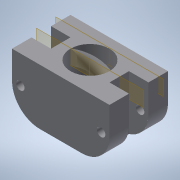
# Autodesk Inventor part: ScrewActuatorGripperCenter
Saved by Autodesk Inventor 2020.1 (Build 241239000, 239)
## iProperties
Created: 2016-10-15
Part Number: ScrewActuatorGripperCenter
Material: Generic
Document SubType Name: Modeling
Designer: Bardo91
Density: 1 g/cm^3
Appearance: Default
Author: Bardo91
Autodesk Inventor part; units mm, degrees
ref_plane "YZ Plane" through (0, 0, 0) normal (1, 0, 0) x (0, 1, 0)
ref_plane "XZ Plane" through (0, 0, 0) normal (0, 1, 0) x (-1, 0, 0)
ref_plane "XY Plane" through (0, 0, 0) normal (0, 0, 1) x (1, 0, 0)
sketch "Sketch1" plane through (0, 0, 0) normal (0, 0, 1) x (1, 0, 0)
  line L0 (0, 0) -> (0, 7)
  line L1 (0, 7) -> (7, 7)
  line L2 (7, 7) -> (7, 0)
  line L3 (7, 0) -> (14, 0)
  line L4 (14, 0) -> (14, 7)
  line L5 (14, 7) -> (21, 7)
  line L6 (21, 7) -> (21, 0)
  line L7 (21, 0) -> (28, 0)
  line L8 (28, 0) -> (28, -7)
  line L9 (28, -7) -> (21, -7)
  line L10 (21, -7) -> (21, -14)
  line L11 (21, -14) -> (28, -14)
  line L12 (28, -14) -> (28, -21)
  line L13 (28, -21) -> (21, -21)
  line L14 (21, -21) -> (21, -28)
  line L15 (21, -28) -> (14, -28)
  line L16 (14, -28) -> (14, -21)
  line L17 (14, -21) -> (7, -21)
  line L18 (7, -21) -> (7, -28)
  line L19 (7, -28) -> (0, -28)
  line L20 (0, -28) -> (0, -21)
  line L21 (0, -21) -> (-7, -21)
  line L22 (-7, -21) -> (-7, -14)
  line L23 (-7, -14) -> (0, -14)
  line L24 (0, -14) -> (0, -7)
  line L25 (0, -7) -> (-7, -7)
  line L26 (-7, -7) -> (-7, 0)
  line L27 (-7, 0) -> (0, 0)
  dimension "d55" = 7
  dimension "d56" = 7
  dimension "d57" = 7
  dimension "d58" = 7
  dimension "d59" = 7
  dimension "d60" = 7
  dimension "d61" = 7
  dimension "d62" = 90
  dimension "d63" = 7
  dimension "d64" = 7
  dimension "d65" = 90
  dimension "d66" = 7
  dimension "d67" = 7
  dimension "d68" = 7
  dimension "d69" = 7
  dimension "d70" = 7
  dimension "d71" = 7
  dimension "d72" = 7
  dimension "d73" = 7
  dimension "d74" = 7
  dimension "d75" = 7
  dimension "d76" = 7
  dimension "d77" = 90
  dimension "d93" = 7
  constraints: 56 end point, 15 perpendicular, 13 point on line, 3 horizontal, 2 vertical
  measures "d55" distance of L0.start L0.end
  measures "d56" distance of L0.end L1.end
  measures "d57" distance of L2.end L3.end
  measures "d58" distance of L3.end L4.end
  measures "d59" distance of L4.end L5.end
  measures "d60" distance of L6.end L7.end
  measures "d61" distance of L7.end L8.end
  measures "d62" angle of L7 L8
  measures "d63" distance of L8.end L9.end
  measures "d64" distance of L9.end L10.end
  measures "d65" angle of L10 L9
  measures "d66" distance of L10.end L11.end
  measures "d67" distance of L11.end L12.end
  measures "d68" distance of L13.end L14.end
  measures "d69" distance of L14.end L15.end
  measures "d70" distance of L16.end L17.end
  measures "d71" distance of L18.end L19.end
  measures "d72" distance of L19.end L20.end
  measures "d73" distance of L20.end L21.end
  measures "d74" distance of L21.end L22.end
  measures "d75" distance of L23.end L24.end
  measures "d76" distance of L24.end L25.end
  measures "d77" angle of L25 L24
  measures "d93" distance of L25.end L26.end
extrude "Extrusion1" add sketch "Sketch1" along normal blind 20
sketch "Sketch6" plane through (0, 0, 20) normal (0, 0, 1) x (1, 0, 0)
  line L0 (14, 0) -> (7, 0) projected
  line L1 (10.5, 0) -> (10.5, -21)
  line L2 (7, -21) -> (14, -21) projected
  circle A0 centre (10.5, -10.5) radius 7
  point P0 (0, 0)
  dimension "d94" = 14
  constraints: 3 midpoint, 2 end point, 1 centre point
  measures "d94" diameter of A0
extrude "Extrusion6" cut sketch "Sketch6" against normal through all
sketch "Sketch7" plane through (-7, -21, 0) normal (0, -1, 0) x (1, 0, 0)
  line L0 (0, 0) -> (0, 10)
  line L1 (0, 0) -> (0, 20) projected
  line L2 (0, 10) -> (3, 10)
  circle A0 centre (3, 10) radius 1.5
  point P0 (7, 0)
  dimension "d83" = 3
  dimension "d84" = 3
  constraints: 4 end point, 1 centre point, 1 coincident, 1 horizontal, 1 midpoint
  measures "d83" distance of L0.end L2.end
  measures "d84" diameter of A0
extrude "Extrusion7" cut sketch "Sketch7" against normal through all
pattern_circular "Circular Pattern3" count 4 over 360 about axis through (10.5, -10.5, 20) along (0, 0, -1) of "Extrusion7"
ref_plane "Work Plane3" through (10.5, -10.5, 20) normal (0, -1, 0) x (1, 0, 0)
ref_plane "Work Plane2" through (10.5, -3.5, 20) normal (0, -1, 0) x (1, 0, 0)
sketch "Sketch10" plane through (10.5, -10.5, 20) normal (0, -1, 0) x (1, 0, 0)
  line L0 (-7, 0) -> (7, 0) projected
  line L1 (-7, 0) -> (-4.5, 0)
  line L2 (-4.5, 0) -> (-4.5, -5)
  line L3 (-4.5, -5) -> (-7, -5)
  line L4 (-7, -5) -> (-7, 0)
  point P0 (-10.5, -20)
  dimension "d100" = 2.5
  dimension "d101" = 5
  constraints: 8 end point, 3 perpendicular, 1 point on line
  measures "d100" distance of L0.start L1.end
  measures "d101" distance of L1.end L2.end
coil "Coil1" sketch "Sketch10" operation add axis through (10.5, -10.5, 20) along (0, 0, -1) pitch 25 turns 0.6 hand right
fillet "Fillet4" radius 2 4 edges at (7.855, -6.8594, 16.25) (14.7797, -9.1094, 8.75) (7.855, -6.8594, 11.25) (14.7797, -9.1094, 3.75)
fillet "Fillet5" radius 10 2 edges at (-7, -17.5, 0) (28, -17.5, 0)
sketch "Sketch11" plane through (0, 0, 0) normal (0, 0, -1) x (-1, 0, 0)
  line L0 (-28, 0) -> (-21, 0) projected
  line L1 (-28, 0) -> (7.1742, 0)
  line L2 (7.1742, 0) -> (7.1742, 7.7318)
  line L3 (7.1742, 7.7318) -> (-28, 7.7318)
  line L4 (-28, 7.7318) -> (-28, 0)
  line L5 (7, -14) -> (7, -21) projected
  line L6 (7, -21) -> (-30.6693, -21)
  line L7 (-30.6693, -21) -> (-30.6693, -32.4769)
  line L8 (-30.6693, -32.4769) -> (7, -32.4769)
  line L9 (7, -32.4769) -> (7, -21)
  point P0 (0, 0)
  constraints: 16 end point, 4 parallel, 2 horizontal, 2 perpendicular
extrude "Extrusion8" cut sketch "Sketch11" against normal up to surface (20 mm away)
equation "\"d55\" = d76"
equation "\"d56\" = d76"
equation "\"d57\" = d76"
equation "\"d58\" = d76"
equation "\"d59\" = d76"
equation "\"d60\" = d61"
equation "\"d61\" = d63"
equation "\"d63\" = d64"
equation "\"d64\" = d66"
equation "\"d66\" = d68"
equation "\"d67\" = d68"
equation "\"d68\" = d69"
equation "\"d70\" = d68"
equation "\"d71\" = d70"
equation "\"d72\" = d70"
equation "\"d73\" = d70"
equation "\"d75\" = d70"
equation "\"d76\" = d70"
equation "\"d93\" = d76"
body "Solid1"
